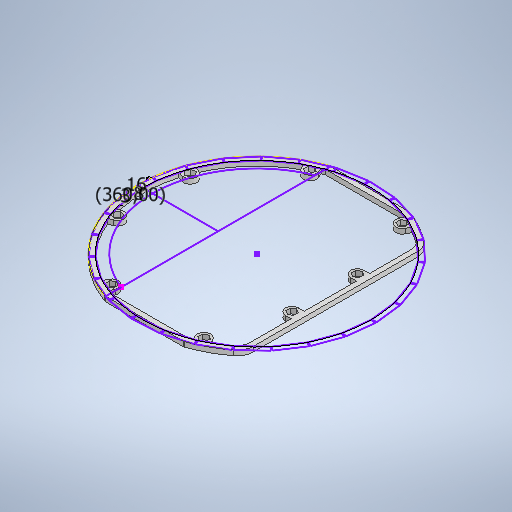
# Autodesk Inventor part: carcasa
Saved by Autodesk Inventor 2025.2 (Build 292293000, 293)
## iProperties
Created: 2025-08-27
Part Number: carcasa
Material: Generic
Document SubType Name: Modeling
Designer: cdavi
Density: 1 g/cm^3
Appearance: Default
Author: cdavi
Autodesk Inventor part; units mm, degrees
ref_plane "YZ Plane" through (0, 0, 0) normal (1, 0, 0) x (0, 1, 0)
ref_plane "XZ Plane" through (0, 0, 0) normal (0, 1, 0) x (-1, 0, 0)
ref_plane "XY Plane" through (0, 0, 0) normal (0, 0, 1) x (1, 0, 0)
sketch "Sketch1" plane through (0, 0, 0) normal (0, 1, 0) x (-1, 0, 0)
  line L0 (23.1517, 65.9375) -> (-23.1517, 65.9375)
  line L1 (0, 0) -> (-48, 0) construction
  line L2 (23.6722, 68.9375) -> (-23.6722, 68.9375)
  line L3 (23.1517, -65.9375) -> (-23.5, -65.9375)
  line L4 (23.6722, -68.9375) -> (-23.6722, -68.9375)
  line L5 (0, 0) -> (0, 68.9375) construction
  line L6 (-45, 48.734) -> (-45, -48.734)
  line L7 (-48, 50.2494) -> (-48, -50.2494)
  arc A0 (-40.8333, -56.8563) -> (-23.5, -65.9375) centre (0, 0) ccw
  arc A1 (-44.0317, -58.2255) -> (-24.3391, -68.823) centre (0, 0) ccw
  arc A2 (24.3391, -68.823) -> (24.3391, 68.823) centre (0, 0) ccw
  arc A3 (-24.3391, 68.823) -> (-44.0317, 58.2255) centre (0, 0) ccw
  arc A4 (23.8326, -65.818) -> (23.8326, 65.818) centre (0, 0) ccw
  arc A5 (-23.8326, 65.818) -> (-40.8333, 56.8563) centre (0, 0) ccw
  arc A6 (-24.3391, -68.823) -> (-23.6722, -68.9375) centre (-23.6722, -66.9375) ccw
  arc A7 (23.6722, -68.9375) -> (24.3391, -68.823) centre (23.6722, -66.9375) ccw
  arc A8 (23.1517, -65.9375) -> (23.8326, -65.818) centre (23.1517, -63.9375) ccw
  arc A9 (23.8326, 65.818) -> (23.1517, 65.9375) centre (23.1517, 63.9375) ccw
  arc A10 (24.3391, 68.823) -> (23.6722, 68.9375) centre (23.6722, 66.9375) ccw
  arc A11 (-23.1517, 65.9375) -> (-23.8326, 65.818) centre (-23.1517, 63.9375) ccw
  arc A12 (-23.6722, 68.9375) -> (-24.3391, 68.823) centre (-23.6722, 66.9375) ccw
  arc A13 (-40.8333, 56.8563) -> (-45, 48.734) centre (-35, 48.734) ccw
  arc A14 (-44.0317, 58.2255) -> (-48, 50.2494) centre (-38, 50.2494) ccw
  arc A15 (-48, -50.2494) -> (-44.0317, -58.2255) centre (-38, -50.2494) ccw
  arc A16 (-45, -48.734) -> (-40.8333, -56.8563) centre (-35, -48.734) ccw
  point P0 (-24.013, 68.9375)
  point P1 (23.5, -65.9375)
  point P2 (24.013, -68.9375)
  point P3 (-24.013, -68.9375)
  point P4 (-48, -55)
  point P5 (-45, 53.619)
  point P6 (-45, -53.619)
  point P7 (-48, 55)
  point P8 (24.013, 68.9375)
  point P9 (23.5, 65.9375)
  point P10 (-23.5, 65.9375)
  dimension "d2" = 65.9375
  dimension "d4" = 3
  dimension "d6" = 45
  dimension "d7" = 3
  dimension "d8" = 2
  dimension "d9" = 10
  dimension "d10" = 70
  dimension "d11" = 73
  dimension "d12" = 70
  dimension "d13" = 73
  constraints: 45 point on circle, 22 tangent, 17 centre point, 16 end point, 11 point on line, 9 equal radius, 4 symmetric about line, 3 vertical, 2 coincident, 2 horizontal, 2 midpoint, 1 parallel
  measures "d2" distance between parallel lines of L1 L0
  measures "d4" distance between parallel lines of L0 L2
  measures "d6" distance between parallel lines of L6 L5
  measures "d7" distance between parallel lines of L7 L6
  measures "d8" radius of A6
  measures "d9" radius of A13
  measures "d10" radius of A4
  measures "d11" radius of A2
  measures "d12" radius of A0
  measures "d13" radius of A1
extrude "Extrusion1" add sketch "Sketch1" along normal blind 65
sketch "Sketch2" plane through (48, 0, 50.2494) normal (1, 0, 0) x (0, 0, -1)
  line L0 (50.2494, 0) -> (50.2494, 65) construction
  line L1 (98.9833, 65) -> (1.5154, 65) projected
  line L2 (0.4263, 38) -> (20.4263, 38)
  line L3 (20.4263, 38) -> (20.4263, 26)
  line L4 (20.4263, 26) -> (0.4263, 26)
  line L5 (0.4263, 26) -> (0.4263, 38)
  line L6 (0, 0) -> (100.4988, 0) projected
  line L7 (-18.5737, 0) -> (-18.5737, 65) projected
  line L8 (100.0724, 38) -> (80.0724, 38)
  line L9 (80.0724, 38) -> (80.0724, 26)
  line L10 (80.0724, 26) -> (100.0724, 26)
  line L11 (100.0724, 26) -> (100.0724, 38)
  dimension "d16" = 26
  dimension "d17" = 19
  dimension "d18" = 12
  dimension "d19" = 20
  constraints: 18 end point, 4 symmetric about line, 2 parallel, 1 horizontal, 1 midpoint, 1 perpendicular
  measures "d16" distance between parallel lines of L6 L4
  measures "d17" distance between parallel lines of L5 L7
  measures "d18" distance of L2.end L3.end
  measures "d19" distance of L2.start L2.end
extrude "Extrusion2" cut sketch "Sketch2" against normal blind 5
sketch "Sketch3" plane through (48, 0, 50.2494) normal (1, 0, 0) x (0, 0, -1)
  line L0 (3.568, 49.2223) -> (17.7975, 43.9952) construction
  line L1 (2.8909, 47.379) -> (17.1204, 42.1519)
  line L2 (18.4746, 45.8385) -> (4.2452, 51.0656)
  arc A0 (4.2452, 51.0656) -> (2.8909, 47.379) centre (3.568, 49.2223) ccw
  arc A1 (17.1204, 42.1519) -> (18.4746, 45.8385) centre (17.7975, 43.9952) ccw
  arc A2 (44.4296, 11.624) -> (34.6921, 2.9774) centre (43.8866, 2.4292) ccw construction
  arc A3 (44.531, 13.3402) -> (32.9759, 3.0797) centre (43.8866, 2.4292) ccw
  arc A4 (44.3283, 9.9077) -> (36.4083, 2.8751) centre (43.8866, 2.4292) ccw
  arc A5 (44.3283, 9.9077) -> (44.531, 13.3402) centre (44.4296, 11.624) ccw
  arc A6 (32.9759, 3.0797) -> (36.4083, 2.8751) centre (34.6921, 2.9774) ccw
  line L3 (50.2494, 0) -> (50.2494, 65) construction
  line L4 (97.6079, 47.379) -> (83.3784, 42.1519)
  line L5 (82.0241, 45.8385) -> (96.2536, 51.0656)
  arc A7 (97.6079, 47.379) -> (96.2536, 51.0656) centre (96.9307, 49.2223) ccw
  arc A8 (82.0241, 45.8385) -> (83.3784, 42.1519) centre (82.7013, 43.9952) ccw
  point P0 (10.6828, 46.6088)
  constraints: 18 point on circle, 12 end point, 9 centre point, 8 tangent, 6 symmetric about line, 1 midpoint, 1 parallel, 2 other
extrude "Extrusion3" [suppressed]
extrude "Extrusion4" add sketch "Sketch1" along normal blind 3 from surface at 65 separate body contours A9 A4 A8 L3 A0 A16 L6 A13 A5 A11 L0 | A10 A2 A7 L4 A6 A1 A15 L7 A14 A3 A12 L2
sketch "Sketch5" plane through (-23.6722, 68, 68.9375) normal (0, 1, 0) x (1, 0, 0)
  circle A0 centre (23.6722, 68.9375) radius 8.5
  circle A1 centre (-6.3278, 68.9375) radius 2.5
  line L0 (31.7963, 66.4375) -> (40.6722, 66.4375)
  line L1 (40.6722, 66.4375) -> (40.6722, 71.4375)
  line L2 (40.6722, 71.4375) -> (31.7963, 71.4375)
  point P0 (40.6722, 68.9375)
  dimension "d26" = 17
  dimension "d27" = 5
  dimension "d31" = 5
  dimension "d32" = 17
  dimension "d47" = 30
  constraints: 6 end point, 2 centre point, 2 horizontal alignment, 2 perpendicular, 2 point on circle, 1 coincident, 1 horizontal, 1 midpoint
  measures "d26" diameter of A0
  measures "d27" diameter of A1
  measures "d31" distance between parallel lines of L2 L0
  measures "d32" distance from line of A0.centre L1
  measures "d47" distance of A0.centre A1.centre
extrude "Extrusion5" cut sketch "Sketch5" against normal through all bodies 2
sketch "Sketch6" plane through (0, 0, 0) normal (0, 1, 0) x (-1, 0, 0)
  circle A0 centre (0, 0) radius 67 construction
  arc A1 (-23.8326, 65.818) -> (-40.8333, 56.8563) centre (0, 0) ccw projected
  arc A2 (-40.8333, 56.8563) -> (-45, 48.734) centre (-35, 48.734) ccw projected
  line L0 (-45, -48.734) -> (-45, 48.734) projected
  arc A3 (-45, -48.734) -> (-40.8333, -56.8563) centre (-35, -48.734) ccw projected
  arc A4 (-40.8333, -56.8563) -> (-23.5, -65.9375) centre (0, 0) ccw projected
  line L1 (23.1517, -65.9375) -> (-23.5, -65.9375) construction
  arc A5 (23.8326, -65.818) -> (23.8326, 65.818) centre (0, 0) ccw projected
  line L2 (-23.1517, 65.9375) -> (23.1517, 65.9375) construction
  line L3 (23.6722, 68.9375) -> (-23.6722, 68.9375) projected
  arc A6 (-24.3391, 68.823) -> (-44.0317, 58.2255) centre (0, 0) ccw projected
  arc A7 (-44.0317, 58.2255) -> (-48, 50.2494) centre (-38, 50.2494) ccw projected
  line L4 (-48, 50.2494) -> (-48, -50.2494) projected
  arc A8 (-48, -50.2494) -> (-44.0317, -58.2255) centre (-38, -50.2494) ccw projected
  arc A9 (-44.0317, -58.2255) -> (-24.3391, -68.823) centre (0, 0) ccw projected
  line L5 (-23.6722, -68.9375) -> (23.6722, -68.9375) projected
  arc A10 (24.3391, -68.823) -> (24.3391, 68.823) centre (0, 0) ccw projected
  arc A11 (-22.7858, 59.8064) -> (-37.3333, 51.9829) centre (0, 0) ccw construction
  arc A12 (-37.3333, 51.9829) -> (-39, 48.734) centre (-35, 48.734) ccw construction
  line L6 (-39, 48.734) -> (-39, -48.734) construction
  arc A13 (-39, -48.734) -> (-37.3333, -51.9829) centre (-35, -48.734) ccw construction
  arc A14 (-37.3333, -51.9829) -> (-22.7858, -59.8064) centre (0, 0) ccw construction
  line L7 (-22.0737, -59.9375) -> (22.0737, -59.9375) construction
  line L8 (-22.0737, 59.9375) -> (22.0737, 59.9375) construction
  arc A15 (22.7858, -59.8064) -> (22.7858, 59.8064) centre (0, 0) ccw construction
  arc A16 (-8.124, -2.5) -> (-8.124, 2.5) centre (0, 0) ccw projected
  line L9 (0, 0) -> (63.1919, 22.2662) construction
  line L10 (0, 0) -> (73, 0) construction
  circle A17 centre (63.1919, 22.2662) radius 2.85 construction
  line L11 (0, 0) -> (0, -67) construction
  circle A18 centre (28.3154, 60.7226) radius 2.85 construction
  line L12 (28.3154, 60.7226) -> (0, 0) construction
  circle A19 centre (-41.5, 20) radius 2.85 construction
  circle A20 centre (-28.3154, 60.7226) radius 2.85 construction
  line L13 (-28.3154, 60.7226) -> (0, 0) construction
  arc A21 (-22.0737, 59.9375) -> (-22.7858, 59.8064) centre (-22.0737, 57.9375) ccw construction
  arc A22 (-22.7858, -59.8064) -> (-22.0737, -59.9375) centre (-22.0737, -57.9375) ccw construction
  arc A23 (22.0737, -59.9375) -> (22.7858, -59.8064) centre (22.0737, -57.9375) ccw construction
  arc A24 (22.7858, 59.8064) -> (22.0737, 59.9375) centre (22.0737, 57.9375) ccw construction
  arc A25 (-24.3391, -68.823) -> (-23.6722, -68.9375) centre (-23.6722, -66.9375) ccw projected
  arc A26 (23.6722, -68.9375) -> (24.3391, -68.823) centre (23.6722, -66.9375) ccw projected
  arc A27 (24.3391, 68.823) -> (23.6722, 68.9375) centre (23.6722, 66.9375) ccw projected
  arc A28 (-23.6722, 68.9375) -> (-24.3391, 68.823) centre (-23.6722, 66.9375) ccw projected
  circle A29 centre (63.1919, -22.2662) radius 2.85 construction
  circle A30 centre (28.3154, -60.7226) radius 2.85 construction
  circle A31 centre (-41.5, -20) radius 2.85 construction
  circle A32 centre (-28.3154, -60.7226) radius 2.85 construction
  line L14 (23.8326, 59.397) -> (23.8326, 65.818)
  line L15 (-23.8326, 59.397) -> (-23.8326, 65.818)
  line L16 (23.8326, 65.818) -> (-23.8326, 65.818)
  line L17 (23.8326, -59.397) -> (23.8326, -65.818)
  line L18 (-23.8326, -59.397) -> (-23.8326, -65.818)
  line L19 (23.8326, -65.818) -> (-23.8326, -65.818)
  circle A33 centre (63.1919, 22.2662) radius 4
  circle A34 centre (28.3154, 60.7226) radius 4
  line L20 (60.3905, 22.7899) -> (62.2448, 24.9542)
  line L21 (62.2448, 24.9542) -> (65.0462, 24.4304)
  line L22 (65.0462, 24.4304) -> (65.9934, 21.7424)
  line L23 (65.9934, 21.7424) -> (64.1391, 19.5782)
  line L24 (64.1391, 19.5782) -> (61.3376, 20.1019)
  line L25 (61.3376, 20.1019) -> (60.3905, 22.7899)
  line L26 (25.9808, 59.0879) -> (25.7324, 61.9271)
  line L27 (25.7324, 61.9271) -> (28.067, 63.5618)
  line L28 (28.067, 63.5618) -> (30.65, 62.3573)
  line L29 (30.65, 62.3573) -> (30.8984, 59.5182)
  line L30 (30.8984, 59.5182) -> (28.5638, 57.8835)
  line L31 (28.5638, 57.8835) -> (25.9808, 59.0879)
  circle A35 centre (-41.5, 20) radius 4
  line L32 (-43.9682, 18.575) -> (-43.9682, 21.425)
  line L33 (-43.9682, 21.425) -> (-41.5, 22.85)
  line L34 (-41.5, 22.85) -> (-39.0318, 21.425)
  line L35 (-39.0318, 21.425) -> (-39.0318, 18.575)
  line L36 (-39.0318, 18.575) -> (-41.5, 17.15)
  line L37 (-41.5, 17.15) -> (-43.9682, 18.575)
  line L38 (-41.5, 24) -> (-45, 24)
  line L39 (-41.5, 16) -> (-45, 16)
  circle A36 centre (-28.3154, 60.7226) radius 4
  line L40 (-28.5638, 57.8835) -> (-30.8984, 59.5182)
  line L41 (-30.8984, 59.5182) -> (-30.65, 62.3573)
  line L42 (-30.65, 62.3573) -> (-28.067, 63.5618)
  line L43 (-28.067, 63.5618) -> (-25.7324, 61.9271)
  line L44 (-25.7324, 61.9271) -> (-25.9808, 59.0879)
  line L45 (-25.9808, 59.0879) -> (-28.5638, 57.8835)
  line L46 (-31.8886, 58.9247) -> (-33.2376, 61.6057)
  circle A37 centre (63.1919, -22.2662) radius 4
  circle A38 centre (28.3154, -60.7226) radius 4
  circle A39 centre (-41.5, -20) radius 4
  line L47 (-41.5, -24) -> (-45, -24)
  line L48 (-41.5, -16) -> (-45, -16)
  circle A40 centre (-28.3154, -60.7226) radius 4
  line L49 (-31.8886, -58.9247) -> (-33.2376, -61.6057)
  line L50 (60.3905, -22.7899) -> (62.2448, -24.9542)
  line L51 (62.2448, -24.9542) -> (65.0462, -24.4304)
  line L52 (65.0462, -24.4304) -> (65.9934, -21.7424)
  line L53 (65.9934, -21.7424) -> (64.1391, -19.5782)
  line L54 (64.1391, -19.5782) -> (61.3376, -20.1019)
  line L55 (61.3376, -20.1019) -> (60.3905, -22.7899)
  line L56 (25.9808, -59.0879) -> (25.7324, -61.9271)
  line L57 (25.7324, -61.9271) -> (28.067, -63.5618)
  line L58 (28.067, -63.5618) -> (30.65, -62.3573)
  line L59 (30.65, -62.3573) -> (30.8984, -59.5182)
  line L60 (30.8984, -59.5182) -> (28.5638, -57.8835)
  line L61 (28.5638, -57.8835) -> (25.9808, -59.0879)
  line L62 (-28.5638, -57.8835) -> (-30.8984, -59.5182)
  line L63 (-30.8984, -59.5182) -> (-30.65, -62.3573)
  line L64 (-30.65, -62.3573) -> (-28.067, -63.5618)
  line L65 (-28.067, -63.5618) -> (-25.7324, -61.9271)
  line L66 (-25.7324, -61.9271) -> (-25.9808, -59.0879)
  line L67 (-25.9808, -59.0879) -> (-28.5638, -57.8835)
  line L68 (-43.9682, -18.575) -> (-43.9682, -21.425)
  line L69 (-43.9682, -21.425) -> (-41.5, -22.85)
  line L70 (-41.5, -22.85) -> (-39.0318, -21.425)
  line L71 (-39.0318, -21.425) -> (-39.0318, -18.575)
  line L72 (-39.0318, -18.575) -> (-41.5, -17.15)
  line L73 (-41.5, -17.15) -> (-43.9682, -18.575)
  line L74 (61.7506, 25.9975) -> (64.5502, 27.0789)
  line L75 (64.408, 18.4555) -> (67.2672, 19.368)
  line L76 (31.8886, 58.9247) -> (33.2376, 61.6057)
  line L77 (61.7506, -25.9975) -> (64.5502, -27.0789)
  line L78 (64.408, -18.4555) -> (67.2672, -19.368)
  line L79 (31.8886, -58.9247) -> (33.2376, -61.6057)
  line L80 (-24.6413, 62.3041) -> (-25.828, 65.0609)
  line L81 (24.6413, 62.3041) -> (25.828, 65.0609)
  line L82 (-24.6413, -62.3041) -> (-25.828, -65.0609)
  line L83 (24.6413, -62.3041) -> (25.828, -65.0609)
  point P0 (-22.4388, -59.9375)
  point P1 (28.3154, 60.7226)
  point P2 (28.3154, 60.7226)
  point P3 (-27.1107, 64.5369)
  point P4 (-27.1107, -64.5369)
  point P5 (27.1107, -64.5369)
  point P6 (27.1107, 64.5369)
  point P7 (-45, 21.9365)
  point P8 (-45, 18.0635)
  point P9 (-32.0117, 62.2515)
  point P10 (32.0117, -62.2515)
  point P11 (66.8707, -20.6956)
  point P12 (65.0736, -25.796)
  point P13 (-32.0117, -62.2515)
  point P14 (-45, -21.9365)
  point P15 (-45, -18.0635)
  point P16 (65.0736, 25.796)
  point P17 (66.8707, 20.6956)
  point P18 (32.0117, 62.2515)
  dimension "d33" = 134
  dimension "d39" = 5.7
  dimension "d34" = 6
  dimension "d35" = 6
  dimension "d36" = 6
  dimension "d37" = 19.41
  dimension "d38" = 25
  dimension "d40" = 20
  dimension "d41" = 3.5
  dimension "d42" = 25
  dimension "d44" = 2
  dimension "d61" = 8
  dimension "d62" = 8
  dimension "d63" = 8
  dimension "d64" = 8
  constraints: 156 end point, 52 symmetric about line, 37 point on circle, 20 centre point, 16 tangent, 10 coincident, 6 perpendicular, 3 equal radius, 3 point on line, 2 parallel, 2 vertical, 93 other
  measures "d34" radial gap between concentric circles of A1 A11
  measures "d35" distance between parallel lines of L2 L8
  measures "d36" radial gap between concentric circles of A5 A15
  measures "d37" angle of L10 L9
  measures "d38" angle of L11 L12
  measures "d40" distance from line of point (-41.5, 20) L10
  measures "d41" distance from line of L0 point (-41.5, 20)
  measures "d42" angle of L11 L13
  measures "d44" radius of A21
  measures "d61" diameter of A33
  measures "d62" diameter of A34
  measures "d63" diameter of A35
  measures "d64" diameter of A36
extrude "Extrusion6" add sketch "Sketch6" against normal blind 3 separate body contours L80 A36 A1 | A36 A1 | A1 A36 | A5 A34 L81 | A36 L46 A1 | A34 A5 | A5 A34 | A5 L76 A34 | A5 A33 L74 | L38 A35 L0 | A33 A5 | A5 A33 | A35 L0 | L0 A35 | A5 L75 A33 | A35 L39 L0 | A5 A37 L78 | L48 A39 L0 | A37 A5 | A5 A37 | A39 L0 | L0 A39 | A5 L77 A37 | A39 L47 L0 | A5 A38 L79 | A38 A5 | A5 A38 | A5 L83 A38 | L49 A40 A4 | A40 A4 | A4 A40 | A40 L82 A4 | A27 A10 A26 L5 A25 A9 A8 L4 A7 A6 A28 L3
sketch "Sketch7" plane through (0, 0, 0) normal (0, 1, 0) x (1, 0, 0)
  line L0 (-23.8326, -69.0001) -> (-23.8326, 69.0001)
  line L1 (-23.8326, -59.397) -> (-23.8326, -65.818) projected
  line L2 (-73, 0) -> (-69.5603, 0)
  line L3 (-69.5603, 0) -> (-69.5603, -8)
  line L4 (-69.5603, 0) -> (-69.5603, 8)
  arc A0 (-24.3391, 68.823) -> (-24.3391, -68.823) centre (0, 0) ccw projected
  line L5 (-69.5603, -8) -> (-72.5603, -8)
  line L6 (-72.5603, -8) -> (-72.5603, 8)
  line L7 (-72.5603, 8) -> (-69.5603, 8)
  line L8 (-65.8404, -23.8261) -> (-68.7595, -24.5179)
  line L9 (-68.7595, -24.5179) -> (-72.4494, -8.9492)
  line L10 (-67.6853, -16.0417) -> (-65.8404, -23.8261)
  line L11 (-67.6853, -16.0417) -> (-69.5302, -8.2574)
  line L12 (-72.4494, -8.9492) -> (-69.5302, -8.2574)
  line L13 (-58.571, -38.3677) -> (-61.2519, -39.7141)
  line L14 (-61.2519, -39.7141) -> (-68.4327, -25.416)
  line L15 (-62.1614, -31.2186) -> (-58.571, -38.3677)
  line L16 (-62.1614, -31.2186) -> (-65.7518, -24.0696)
  line L17 (-68.4327, -25.416) -> (-65.7518, -24.0696)
  line L18 (-48.144, -50.8409) -> (-50.4421, -52.7692)
  line L19 (-50.4421, -52.7692) -> (-60.7267, -40.5125)
  line L20 (-53.2863, -44.7125) -> (-48.144, -50.8409)
  line L21 (-53.2863, -44.7125) -> (-58.4286, -38.5842)
  line L22 (-60.7267, -40.5125) -> (-58.4286, -38.5842)
  line L23 (-35.1216, -60.5732) -> (-36.913, -62.9796)
  line L24 (-36.913, -62.9796) -> (-49.747, -53.425)
  line L25 (-41.5385, -55.7959) -> (-35.1216, -60.5732)
  line L26 (-41.5385, -55.7959) -> (-47.9555, -51.0187)
  line L27 (-49.747, -53.425) -> (-47.9555, -51.0187)
  line L28 (-20.2057, -67.04) -> (-21.3939, -69.7947)
  line L29 (-21.3939, -69.7947) -> (-36.0854, -63.4574)
  line L30 (-27.5514, -63.8714) -> (-20.2057, -67.04)
  line L31 (-27.5514, -63.8714) -> (-34.8972, -60.7028)
  line L32 (-36.0854, -63.4574) -> (-34.8972, -60.7028)
  line L33 (-4.2006, -69.8927) -> (-4.7215, -72.8472)
  line L34 (-4.7215, -72.8472) -> (-20.4784, -70.0688)
  line L35 (-12.079, -68.5035) -> (-4.2006, -69.8927)
  line L36 (-12.079, -68.5035) -> (-19.9575, -67.1144)
  line L37 (-20.4784, -70.0688) -> (-19.9575, -67.1144)
  line L38 (12.031, -68.9775) -> (12.2055, -71.9724)
  line L39 (12.2055, -71.9724) -> (-3.7675, -72.9027)
  line L40 (4.0446, -69.4426) -> (12.031, -68.9775)
  line L41 (4.0446, -69.4426) -> (-3.9419, -69.9078)
  line L42 (-3.7675, -72.9027) -> (-3.9419, -69.9078)
  line L43 (27.614, -64.3436) -> (28.4745, -67.2176)
  line L44 (28.4745, -67.2176) -> (13.1466, -71.8065)
  line L45 (19.9501, -66.6381) -> (27.614, -64.3436)
  line L46 (19.9501, -66.6381) -> (12.2862, -68.9325)
  line L47 (13.1466, -71.8065) -> (12.2862, -68.9325)
  line L48 (41.7084, -56.241) -> (43.2084, -58.8391)
  line L49 (43.2084, -58.8391) -> (29.352, -66.8391)
  line L50 (34.7802, -60.241) -> (41.7084, -56.241)
  line L51 (34.7802, -60.241) -> (27.852, -64.241)
  line L52 (29.352, -66.8391) -> (27.852, -64.241)
  line L53 (53.5542, -45.1064) -> (55.6129, -47.2885)
  line L54 (55.6129, -47.2885) -> (43.9749, -58.2684)
  line L55 (47.7352, -50.5963) -> (53.5542, -45.1064)
  line L56 (47.7352, -50.5963) -> (41.9162, -56.0863)
  line L57 (43.9749, -58.2684) -> (41.9162, -56.0863)
  line L58 (62.5129, -31.5401) -> (65.0193, -33.1886)
  line L59 (65.0193, -33.1886) -> (56.2272, -46.5564)
  line L60 (58.1168, -38.224) -> (62.5129, -31.5401)
  line L61 (58.1168, -38.224) -> (53.7207, -44.9079)
  line L62 (56.2272, -46.5564) -> (53.7207, -44.9079)
  line L63 (68.1015, -16.2735) -> (70.9206, -17.2995)
  line L64 (70.9206, -17.2995) -> (65.4482, -32.3346)
  line L65 (65.3653, -23.791) -> (68.1015, -16.2735)
  line L66 (65.3653, -23.791) -> (62.6292, -31.3086)
  line L67 (65.4482, -32.3346) -> (62.6292, -31.3086)
  line L68 (70.0187, -0.1296) -> (72.9984, -0.4778)
  line L69 (72.9984, -0.4778) -> (71.1409, -16.3696)
  line L70 (69.09, -8.0755) -> (70.0187, -0.1296)
  line L71 (69.09, -8.0755) -> (68.1612, -16.0214)
  line L72 (71.1409, -16.3696) -> (68.1612, -16.0214)
  line L73 (68.1612, 16.0214) -> (71.1409, 16.3696)
  line L74 (71.1409, 16.3696) -> (72.9984, 0.4778)
  line L75 (69.09, 8.0755) -> (68.1612, 16.0214)
  line L76 (69.09, 8.0755) -> (70.0187, 0.1296)
  line L77 (72.9984, 0.4778) -> (70.0187, 0.1296)
  line L78 (62.6292, 31.3086) -> (65.4482, 32.3346)
  line L79 (65.4482, 32.3346) -> (70.9206, 17.2995)
  line L80 (65.3653, 23.791) -> (62.6292, 31.3086)
  line L81 (65.3653, 23.791) -> (68.1015, 16.2735)
  line L82 (70.9206, 17.2995) -> (68.1015, 16.2735)
  line L83 (53.7207, 44.9079) -> (56.2272, 46.5564)
  line L84 (56.2272, 46.5564) -> (65.0193, 33.1886)
  line L85 (58.1168, 38.224) -> (53.7207, 44.9079)
  line L86 (58.1168, 38.224) -> (62.5129, 31.5401)
  line L87 (65.0193, 33.1886) -> (62.5129, 31.5401)
  line L88 (41.9162, 56.0863) -> (43.9749, 58.2684)
  line L89 (43.9749, 58.2684) -> (55.6129, 47.2885)
  line L90 (47.7352, 50.5963) -> (41.9162, 56.0863)
  line L91 (47.7352, 50.5963) -> (53.5542, 45.1064)
  line L92 (55.6129, 47.2885) -> (53.5542, 45.1064)
  line L93 (27.852, 64.241) -> (29.352, 66.8391)
  line L94 (29.352, 66.8391) -> (43.2084, 58.8391)
  line L95 (34.7802, 60.241) -> (27.852, 64.241)
  line L96 (34.7802, 60.241) -> (41.7084, 56.241)
  line L97 (43.2084, 58.8391) -> (41.7084, 56.241)
  line L98 (12.2862, 68.9325) -> (13.1466, 71.8065)
  line L99 (13.1466, 71.8065) -> (28.4745, 67.2176)
  line L100 (19.9501, 66.6381) -> (12.2862, 68.9325)
  line L101 (19.9501, 66.6381) -> (27.614, 64.3436)
  line L102 (28.4745, 67.2176) -> (27.614, 64.3436)
  line L103 (-3.9419, 69.9078) -> (-3.7675, 72.9027)
  line L104 (-3.7675, 72.9027) -> (12.2055, 71.9724)
  line L105 (4.0446, 69.4426) -> (-3.9419, 69.9078)
  line L106 (4.0446, 69.4426) -> (12.031, 68.9775)
  line L107 (12.2055, 71.9724) -> (12.031, 68.9775)
  line L108 (-19.9575, 67.1144) -> (-20.4784, 70.0688)
  line L109 (-20.4784, 70.0688) -> (-4.7215, 72.8472)
  line L110 (-12.079, 68.5035) -> (-19.9575, 67.1144)
  line L111 (-12.079, 68.5035) -> (-4.2006, 69.8927)
  line L112 (-4.7215, 72.8472) -> (-4.2006, 69.8927)
  line L113 (-34.8972, 60.7028) -> (-36.0854, 63.4574)
  line L114 (-36.0854, 63.4574) -> (-21.3939, 69.7947)
  line L115 (-27.5514, 63.8714) -> (-34.8972, 60.7028)
  line L116 (-27.5514, 63.8714) -> (-20.2057, 67.04)
  line L117 (-21.3939, 69.7947) -> (-20.2057, 67.04)
  line L118 (-47.9555, 51.0187) -> (-49.747, 53.425)
  line L119 (-49.747, 53.425) -> (-36.913, 62.9796)
  line L120 (-41.5385, 55.7959) -> (-47.9555, 51.0187)
  line L121 (-41.5385, 55.7959) -> (-35.1216, 60.5732)
  line L122 (-36.913, 62.9796) -> (-35.1216, 60.5732)
  line L123 (-58.4286, 38.5842) -> (-60.7267, 40.5125)
  line L124 (-60.7267, 40.5125) -> (-50.4421, 52.7692)
  line L125 (-53.2863, 44.7125) -> (-58.4286, 38.5842)
  line L126 (-53.2863, 44.7125) -> (-48.144, 50.8409)
  line L127 (-50.4421, 52.7692) -> (-48.144, 50.8409)
  line L128 (-65.7518, 24.0696) -> (-68.4327, 25.416)
  line L129 (-68.4327, 25.416) -> (-61.2519, 39.7141)
  line L130 (-62.1614, 31.2186) -> (-65.7518, 24.0696)
  line L131 (-62.1614, 31.2186) -> (-58.571, 38.3677)
  line L132 (-61.2519, 39.7141) -> (-58.571, 38.3677)
  line L133 (-69.5302, 8.2574) -> (-72.4494, 8.9492)
  line L134 (-72.4494, 8.9492) -> (-68.7595, 24.5179)
  line L135 (-67.6853, 16.0417) -> (-69.5302, 8.2574)
  line L136 (-67.6853, 16.0417) -> (-65.8404, 23.8261)
  line L137 (-68.7595, 24.5179) -> (-65.8404, 23.8261)
  line L138 (-23.8326, 0) -> (-73, 0)
  arc A1 (-23.8326, 59.397) -> (-23.8326, -59.397) centre (0, 0) ccw
  arc A2 (-20.4784, 70.0688) -> (-20.4784, -70.0688) centre (0, 0) ccw
  dimension "d49" = 8
  dimension "d51" = 3
  dimension "d52" = 16
  dimension "d55" = 360
  constraints: 277 end point, 8 point on circle, 2 centre point, 2 perpendicular, 2 point on line, 1 coincident, 1 collinear, 1 horizontal, 1 midpoint, 271 other
  measures "d49" distance of L2.end L3.end
  measures "d51" distance of L3.end L5.end
  measures "d52" distance of L5.end L6.end
body "Solid1"
body "Solid2"
body "Solid3"
